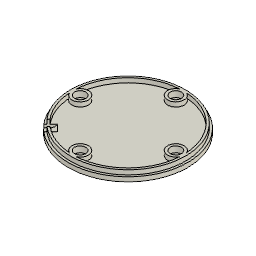
Top_cover (Autodesk Fusion 360 design; units mm, degrees)
part number: 2026-05-20-15-10-24-517
Autodesk Fusion 360 part; units mm, degrees
sketch "Sketch1" plane through (0, 0, 0) normal (0, 0, 1) x (1, 0, 0)
  circle A0 centre (0, 0) radius 40
  circle A1 centre (0, 0) radius 38.5
  dimension "d1" = 80
  dimension "d2" = 77
  constraint coincident A0.centre A1.centre
  constraint concentric A0 A1
  measures "d1" diameter of A0
  measures "d2" diameter of A1
extrude "Extrude1" add sketch "Sketch1" along normal blind 3 contours A0 | A1
extrude "Extrude2" add sketch "Sketch1" along normal blind 3 from surface at 3 contours A1
sketch "Sketch2" plane through (0, 0, 6) normal (0, 0, 1) x (-1, 0, 0)
  circle A0 centre (0, 0) radius 38.5
  circle A1 centre (0, 0) radius 37
  dimension "d8" = 74
  constraint coincident A0.centre A1.centre
  measures "d8" diameter of A1
extrude "Extrude3" cut sketch "Sketch2" against normal blind 3 contours A1
ref_plane "WorkPlane3" through (0, 0, 0) normal (-0.707107, 0.707107, 0) x (0, 0, 1)
sketch "Sketch3" plane through (0, 0, 0) normal (-0.707107, 0.707107, 0) x (0.707107, 0.707107, 0)
  line L0 (-38.5, -6) -> (38.5, -6)
  line L1 (38.5, -3) -> (-38.5, -3)
  line L2 (-40, -3) -> (40, -3)
  line L3 (-40, 0) -> (40, 0)
  line L4 (-40, -3) -> (-40, -1)
  line L5 (-40, -1) -> (-36.546, -1)
  line L6 (-40, -3) -> (-33.385, -3)
  arc A0 (-33.385, -3) -> (-36.546, -1) centre (-36.7574, -4.8322) ccw
  line L7 (-38.5, -6) -> (-36.5, -6)
  line L8 (-36.5, -6) -> (-36.5, -3)
  line L9 (-36.5, -3) -> (-38.5, -3)
  line L10 (-38.5, -3) -> (-38.5, -6)
  dimension "d11" = 2
  dimension "d12" = 3.454
  dimension "d13" = 6.615
  dimension "d14" = 3.838
  dimension "d15" = 3
  dimension "d16" = 2
  constraint coincident L2.start L4.start
  constraint perpendicular L2 L4
  constraint perpendicular L4 L5
  constraint perpendicular L4 L6
  constraint horizontal L7
  constraint vertical L8
  constraint horizontal L9
  constraint vertical L10
  constraint coincident L1.end L9.end
  measures "d11" distance of L2.start L4.end
  measures "d12" distance of L4.end L5.end
  measures "d13" distance of L2.start L6.end
  measures "d14" radius of A0
  measures "d15" distance of L0.start L1.end
  measures "d16" distance of L0.start L7.end
extrude "Extrude4" cut sketch "Sketch3" along normal mid plane 6
sketch "Sketch4" plane through (0, 0, 6) normal (0, 0, 1) x (-1, 0, 0)
  line L0 (23.9555, 28.1981) -> (25.0195, 29.2622)
  arc A0 (25.0195, 29.2622) -> (29.2622, 25.0195) centre (0, 0) ccw
  line L1 (29.2622, 25.0195) -> (28.1981, 23.9555)
  arc A1 (23.9555, 28.1981) -> (28.1981, 23.9555) centre (0, 0) ccw
  arc A2 (23.9555, 28.1981) -> (28.1981, 23.9555) centre (0, 0) ccw
  circle A3 centre (0, -32) radius 5.5
  circle A4 centre (0, -32) radius 3.75
  dimension "d19" = 11
  dimension "d20" = 7.5
  dimension "d23" = 32
  constraint vertical A0.centre A3.centre
  constraint concentric A3 A4
  measures "d19" diameter of A3
  measures "d20" diameter of A4
  measures "d23" distance of A0.centre A3.centre
extrude "Extrude5" add sketch "Sketch4" against normal blind 3 contours A1 A2 A3 | A1 A2 A3 | A4
extrude "Extrude6" cut sketch "Sketch4" against normal blind 4 contours A4
sketch "Sketch5" plane through (0, 0, 0) normal (0, 0, -1) x (1, 0, 0)
  circle A0 centre (0, 0) radius 40
  circle A1 centre (0, -32) radius 3.75
  circle A2 centre (0, -32) radius 3
  dimension "d26" = 6
  constraint concentric A1 A2
  measures "d26" diameter of A2
ref_plane "WorkPlane1" through (0, 0, 2) normal (0, 0, -1) x (1, 0, 0)
sketch "Sketch6" plane through (0, 0, 2) normal (0, 0, -1) x (-1, 0, 0)
  circle A0 centre (0, 32) radius 1.6
  point P0 (0, 32)
  dimension "d29" = 3.2
  constraint vertical P0 A0.centre
  constraint coincident P0 A0.centre
  measures "d29" diameter of A0
loft "Loft1" cut profiles "Sketch5", "Sketch6" section 1 contours A2 section 2
pattern_circular "C-Pattern1" count 4 over 360 about axis through (0, 0, 1.75) along (0, 0, 1) of "Extrude5", "Extrude6", "Loft1"
move_body "Move1" [suppressed]
equation "d2 = ( 38.5 * 2 ) * 1 mm"
equation "d8 = ( 37 * 2 ) * 1 mm"
